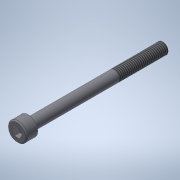
# Autodesk Inventor part: SCREW,SOCKET HD,P,12.9,M5X0.8X60MM
Saved by Autodesk Inventor 2022.4 (Build 264492000, 492)
## iProperties
Category: _
Manager: 100-21762
Created: 2022-12-05
Part Number: SCREW,SOCKET HD,P,12.9,M5X0.8X60MM
Checked By: 0003781382
Engr Approved By: R
User Status: Released
Material: Steel, MS
Description: SCREW, SOCKET HD, P, 12.9, M5X0.8X60MM
Document SubType Name: Modeling
Mfg Approved By: Stephen.Oerton
Designer: Clint.Matte
Manufacturer: Standard
Standards Organization: Custom
Density: 7.86 g/cm^3
Appearance: Metal-Steel
Mass: 11.1887 g
Surface Area: 12.136 cm^2
Volume: 1.4235 cm^3
CN_MASS: 0.01
CN_SERVICEABLE: _
FIRST_DESCRIPTION: _
SECOND_DESCRIPTION: _
THIRD_DESCRIPTION: _
ModelCat: Uncategorized
PTC_WM_ITERATION: 2
PTC_WM_ORGANIZATION_ID: CLWC
PTC_WM_LIFECYCLE: CLWC_CAD_LC
Subject: _
Author: Clint.Matte
Keywords: -
Revision Number: A
Autodesk Inventor part; units mm, degrees
ref_plane "YZ Plane" through (0, 0, 0) normal (1, 0, 0) x (0, 1, 0)
ref_plane "XZ Plane" through (0, 0, 0) normal (0, 1, 0) x (-1, 0, 0)
ref_plane "XY Plane" through (0, 0, 0) normal (0, 0, 1) x (1, 0, 0)
sketch "Sketch3" plane through (0, 0, 0) normal (0, 0, 1) x (1, 0, 0)
  circle A0 centre (0, 0) radius 2.5
  dimension "Diameter" = 5
  constraints: 1 centre point, 1 coincident
  measures "Diameter" diameter of A0
extrude "Extrusion1" add sketch "Sketch3" against normal blind 60
sketch "Sketch4" plane through (0, 0, 0) normal (0, 0, 1) x (1, 0, 0)
  circle A0 centre (0, 0) radius 2.5 projected
  circle A1 centre (0, 0) radius 4.25
  dimension "Head_Diameter" = 8.5
  constraints: 1 centre point, 1 coincident
  measures "Head_Diameter" diameter of A1
extrude "Extrusion2" add sketch "Sketch4" along normal blind 5 contours A0 | A1
sketch "Sketch5" plane through (0, 0, 5) normal (0, 0, 1) x (1, 0, 0)
  circle A0 centre (0, 0) radius 4.25 projected
  line L0 (2.3094, 0) -> (1.1547, -2)
  line L1 (1.1547, -2) -> (-1.1547, -2)
  line L2 (-1.1547, -2) -> (-2.3094, 0)
  line L3 (-2.3094, 0) -> (-1.1547, 2)
  line L4 (-1.1547, 2) -> (1.1547, 2)
  line L5 (1.1547, 2) -> (2.3094, 0)
  line L6 (0, 0) -> (2.3094, 0) construction
  dimension "Hex_Width" = 4
  constraints: 14 end point, 1 coincident, 1 horizontal, 13 other
  measures "Hex_Width" distance between parallel lines of L1 L4
extrude "Extrusion3" cut sketch "Sketch5" against normal blind 2.5 contours L0 L1 L2 L3 L4 L5
thread "Thread1" size "M5x0.8" class "4g6g" standard "ANSI Metric M Profile" length 22
chamfer "Chamfer1" distance 0.5 angle 45 1 edges at (-4.25, 0, 5)
chamfer "Chamfer2" distance 0.25 angle 45 1 edges at (-2.5, 0, -60)
equation "\"d14\" = 0.5 * Chamfer"
equation "\"Chamfer\" = 0.5"
body "Solid1"
